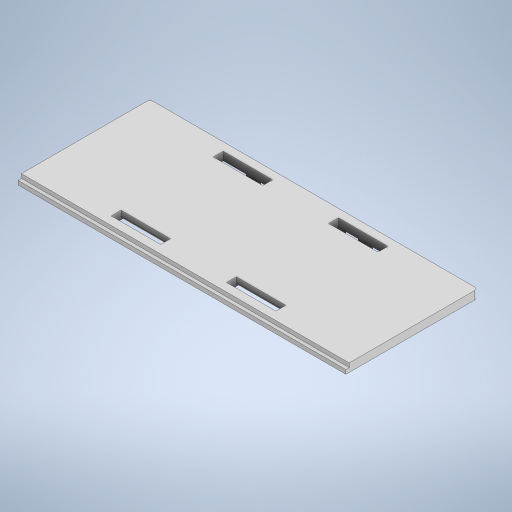
# Autodesk Inventor part: Kryt těla
Saved by Autodesk Inventor 2023 (Build 270158000, 158)
## iProperties
Created: 2023-03-18
Part Number: Kryt těla
Material: Všeobecné
Document SubType Name: Modeling
Designer: jaryj
Density: 1 g/cm^3
Appearance: Výchozí
Author: jaryj
Autodesk Inventor part; units mm, degrees
ref_plane "YZ Plane" through (0, 0, 0) normal (1, 0, 0) x (0, 1, 0)
ref_plane "XZ Plane" through (0, 0, 0) normal (0, 1, 0) x (-1, 0, 0)
ref_plane "XY Plane" through (0, 0, 0) normal (0, 0, 1) x (1, 0, 0)
sketch "Náčrt1" plane through (0, 0, 0) normal (0, 1, 0) x (-1, 0, 0)
  line L0 (0, 0) -> (49.75, 0)
  line L1 (49.75, 0) -> (49.75, -40)
  line L2 (49.75, -40) -> (0, -40)
  line L3 (0, -40) -> (0, 0)
  line L4 (0, -1) -> (49.75, -1)
  line L5 (18, -37) -> (16, -37)
  line L6 (18, -37) -> (18, -39.9)
  line L7 (18, -39.9) -> (16, -39.9)
  line L8 (16, -39.9) -> (16, -37)
  line L9 (5.25, -40) -> (5.25, -36)
  line L10 (5.25, -36) -> (9.75, -36)
  line L11 (9.75, -36) -> (9.75, -40)
  dimension "d0" = 40
  dimension "d1" = 49.75
  dimension "d2" = 1
  dimension "d5" = 3
  dimension "d16" = 0.1
  dimension "d17" = 31.75
  dimension "d18" = 2
  dimension "d28" = 4.5
  dimension "d29" = 4
  dimension "d30" = 5.25
  constraints: 24 end point, 7 perpendicular, 4 point on line, 2 parallel, 1 horizontal, 1 vertical
  measures "d0" distance of L2.end L0.start
  measures "d1" distance of L1.end L2.end
  measures "d2" distance between parallel lines of L0 L4
  measures "d5" distance between parallel lines of L2 L5
  measures "d16" distance between parallel lines of L2 L7
  measures "d17" distance from line of L1 L5.start
  measures "d18" distance of L5.start L5.end
  measures "d28" distance of L9.end L10.end
  measures "d29" distance of L10.end L11.end
  measures "d30" distance between parallel lines of L3 L9
extrude "Vysunutí1" add sketch "Náčrt1" along normal blind 2.5 contours L4 L1 L2 L11 L10 L9 L3 | L9 L10 L11 L2 | L6 L7 L8 L5
extrude "Vysunutí2" add sketch "Náčrt1" along normal blind 1.25 contours L0 L1 L4 L3
extrude "Vysunutí3" add sketch "Náčrt1" against normal blind 12.5 contours L6 L7 L8 L5
sketch "Náčrt3" plane through (-16, 0, -39.9) normal (0, 0, -1) x (-1, 0, 0)
  line L0 (0, 0) -> (0, -12.5) projected
  line L1 (0, -12.5) -> (2, -12.5) projected
  line L2 (2, 0) -> (2, -12.5) projected
  line L3 (0, 0) -> (0, -12.5) projected
  line L4 (0, -10.6) -> (2, -10.6)
  line L5 (2, 0) -> (2, -12.5) projected
  point P0 (-16, 0)
  point P1 (2, -10.6)
  point P2 (0, -10.6)
  dimension "d19" = 1.9
  constraints: 2 end point, 2 point on line, 1 perpendicular
  measures "d19" distance between parallel lines of L4 L1
extrude "Vysunutí5" add sketch "Náčrt3" along normal blind 5
fillet "Zaoblení1" radius 1 1 edges at (-49.75, 1.25, -40)
extrude "Vysunutí6" add sketch "Náčrt1" against normal blind 8 contours L9 L10 L11 L2
sketch "Náčrt7" plane through (-5.25, -8, -36) normal (1, 0, 0) x (0, 0, -1)
  line L0 (0, 8) -> (0, 0) projected
  line L1 (0, 0) -> (4, 0) projected
  line L2 (4, 8) -> (4, 0) projected
  line L3 (0, 8) -> (0, 0) projected
  line L4 (0, 2) -> (4, 2)
  line L5 (4, 8) -> (4, 0) projected
  point P0 (-36, 8)
  dimension "d36" = 2
  constraints: 2 end point, 2 point on line, 1 perpendicular
  measures "d36" distance between parallel lines of L1 L4
extrude "Vysunutí8" add sketch "Náčrt7" along normal up to surface (5.25 mm away)
sketch "Náčrt8" plane through (0, 0, -40) normal (0, 0, -1) x (-1, 0, 0)
  line L0 (9.75, 0) -> (9.75, -8) projected
  line L1 (5.25, -6) -> (0, -6) projected
  point P0 (0, 0)
  point P1 (7.5, -3)
  dimension "d46" = 2.25
  dimension "d47" = 3
  measures "d46" distance from line of L0 point (7.5, -3)
  measures "d47" distance from line of L1 point (7.5, -3)
hole "Díra1" at (-7.5, -3, -40) direction (0, 0, 1) diameter 2 end through all
sketch "Náčrt9" plane through (0, 2.5, 0) normal (0, 1, 0) x (1, 0, 0)
  line L0 (-25, 6.5) -> (-10, 6.5)
  line L1 (-10, 6.5) -> (-10, 3.5)
  line L2 (-10, 3.5) -> (-25, 3.5)
  line L3 (-25, 3.5) -> (-25, 6.5)
  line L4 (-25, 37.5) -> (-10, 37.5)
  line L5 (-10, 37.5) -> (-10, 34.5)
  line L6 (-10, 34.5) -> (-25, 34.5)
  line L7 (-25, 34.5) -> (-25, 37.5)
  line L8 (-25, 37.5) -> (-25, 40) construction
  line L9 (-9.75, 40) -> (-48.75, 40) projected
  line L10 (-25, 3.5) -> (-25, 1) construction
  line L11 (-49.75, 1) -> (0, 1) projected
  line L12 (0, 40) -> (0, 1) projected
  point P0 (0, 0)
  dimension "d48" = 3
  dimension "d49" = 3
  dimension "d50" = 15
  dimension "d51" = 28
  dimension "d52" = 25
  constraints: 20 end point, 5 point on line, 4 parallel, 2 horizontal, 2 perpendicular, 1 collinear, 1 vertical
  measures "d48" distance of L6.end L4.start
  measures "d49" distance of L2.end L0.start
  measures "d50" distance of L4.start L4.end
  measures "d51" distance between parallel lines of L0 L6
  measures "d52" distance between parallel lines of L12 L7
extrude "Vysunutí9" cut sketch "Náčrt9" against normal through all
fillet "Zaoblení2" radius 1 2 edges at (-17.5, 0, -6.5) (-17.5, 0, -34.5)
mirror "Zrcadlit2" about plane through (0, 0, -40) normal (1, 0, 0)
